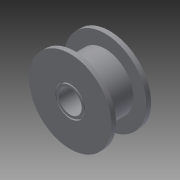
# Autodesk Inventor part: Wheel
Saved by Autodesk Inventor 2015 (Build 190159000, 159)
## iProperties
Created: 2017-01-30
Part Number: Wheel
Material: Generic
Document SubType Name: Modeling
Designer: Ernest
Density: 1 g/cm^3
Appearance: Default
Author: Ernest
Autodesk Inventor part; units mm, degrees
ref_plane "YZ Plane" through (0, 0, 0) normal (1, 0, 0) x (0, 1, 0)
ref_plane "XZ Plane" through (0, 0, 0) normal (0, 1, 0) x (-1, 0, 0)
ref_plane "XY Plane" through (0, 0, 0) normal (0, 0, 1) x (1, 0, 0)
sketch "Sketch1" plane through (0, 0, 0) normal (0, 1, 0) x (-1, 0, 0)
  circle A0 centre (0, 0) radius 2.5
  circle A1 centre (0, 0) radius 8.95
  circle A2 centre (0, 0) radius 6.1
  dimension "d0" = 5
  dimension "d1" = 17.9
  dimension "d2" = 12.2
  constraints: 3 centre point, 3 coincident
  measures "d0" diameter of A0
  measures "d1" diameter of A1
  measures "d2" diameter of A2
extrude "Extrusion1" add sketch "Sketch1" along normal blind 1 contours A1 | A2
extrude "Extrusion2" add sketch "Sketch1" along normal blind 7.6 contours A2
sketch "Sketch2" plane through (0, 7.6, 0) normal (0, 1, 0) x (1, 0, 0)
  circle A0 centre (0, 0) radius 8.95 projected
  circle A1 centre (0, 0) radius 2.5
  constraints: 1 centre point, 1 coincident
extrude "Extrusion3" add sketch "Sketch2" along normal blind 1
sketch "Sketch3" plane through (0, 0, 0) normal (0, -1, 0) x (1, 0, 0)
  circle A0 centre (0, 0) radius 3
  circle A1 centre (0, 0) radius 3.25
  dimension "d9" = 6
  dimension "d10" = 6.5
  constraints: 2 centre point, 2 coincident
  measures "d9" diameter of A0
  measures "d10" diameter of A1
sketch "Sketch4" plane through (0, 8.6, 0) normal (0, 1, 0) x (1, 0, 0)
  circle A0 centre (0, 0) radius 3
  circle A1 centre (0, 0) radius 3.25
  dimension "d11" = 6
  dimension "d12" = 6.5
  constraints: 2 centre point, 2 coincident
  measures "d11" diameter of A0
  measures "d12" diameter of A1
extrude "Extrusion4" cut sketch "Sketch4" against normal blind 0.5
extrude "Extrusion5" cut sketch "Sketch3" against normal blind 0.5
body "Solid1"
